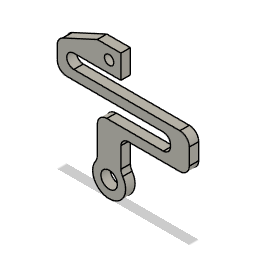
_VEER.274ef9a5-93d1-4273-a178-3e04e85e3114 (Autodesk Fusion 360 design; units mm, degrees)
Autodesk Fusion 360 part; units mm, degrees
sketch "Sketch1" plane through (0, 0, 0) normal (0, 0, 1) x (1, 0, 0)
  line L0 (2.5, 19.5) -> (2.5, 24.5)
  line L1 (-8.5, 21.7171) -> (-8.5, 21.7081)
  line L2 (2.5, 19.5) -> (2.5, 24.5)
  circle A0 centre (0, 0) radius 1.75
  circle A1 centre (0, 22) radius 1
  line L3 (0, 19.5812) -> (0, -19.5812) construction
  line L4 (2.5, 0) -> (-2.5, 0)
  line L5 (-2.5, 3.1623) -> (-2.5, 9)
  line L6 (-0.5, 11) -> (2.5, 11)
  line L7 (2.5, 7.5) -> (2.5, 3.1623)
  line L8 (2.5, 0) -> (-2.5, 11) construction
  line L9 (-2.5, 0) -> (2.5, 11) construction
  line L10 (-0.5, 11) -> (11.5, 11)
  line L11 (17, 11) -> (17, 9)
  line L12 (15, 9) -> (4, 9)
  line L13 (-2.5, 9) -> (-2.5, 11)
  line L14 (17, 9) -> (13, 9)
  line L15 (13, 12.5) -> (13, 13)
  line L16 (13, 16.5) -> (17, 16.5)
  line L17 (17, 14.5) -> (17, 11)
  line L18 (15, 16.5) -> (-7.5, 16.5)
  line L19 (-9, 14.5) -> (11.5, 14.5)
  line L20 (17, 14.5) -> (17, 16.5)
  line L21 (2.5, 19.5) -> (-2.5, 19.5)
  line L22 (-2.5, 19.5) -> (-2.5, 24.5)
  line L23 (-2.5, 24.5) -> (2.5, 24.5)
  line L24 (2.5, 24.5) -> (2.5, 19.5)
  line L25 (2.5, 19.5) -> (-2.5, 24.5) construction
  line L26 (-2.5, 19.5) -> (2.5, 24.5) construction
  line L27 (2.5, 19.5) -> (-7.5, 19.5)
  line L28 (-2.5, 21.5) -> (2.5, 21.5)
  line L29 (2.5, 21.5) -> (2.5, 19.5)
  line L30 (-9, 18) -> (-11, 18)
  line L31 (-11, 16.5) -> (-11, 19.2973)
  line L32 (-2.5, 24.5) -> (-9.8381, 21.1132)
  arc A2 (-7.5, 19.5) -> (-9, 18) centre (-7.5, 18) ccw
  arc A3 (-9, 18) -> (-7.5, 16.5) centre (-7.5, 18) ccw
  arc A4 (13, 13) -> (11.5, 14.5) centre (11.5, 13) ccw
  arc A5 (11.5, 11) -> (13, 12.5) centre (11.5, 12.5) ccw
  arc A6 (4, 9) -> (2.5, 7.5) centre (4, 7.5) ccw
  arc A7 (-11, 16.5) -> (-9, 14.5) centre (-9, 16.5) ccw
  arc A8 (17, 14.5) -> (15, 16.5) centre (15, 14.5) ccw
  arc A9 (15, 9) -> (17, 11) centre (15, 11) ccw
  arc A10 (-9.8381, 21.1132) -> (-11, 19.2973) centre (-9, 19.2973) ccw
  arc A11 (-0.5, 11) -> (-2.5, 9) centre (-0.5, 9) ccw
  arc A12 (-0.9716, 3.3624) -> (-2.5, 2.4495) centre (0, 0) ccw
  arc A13 (-2.8636, 2.0124) -> (2.8636, 2.0124) centre (0, 0) ccw
  arc A14 (0.9716, 3.3624) -> (-0.9716, 3.3624) centre (0, 0) ccw
  arc A15 (2.5, 2.4495) -> (0.9716, 3.3624) centre (0, 0) ccw
  arc A16 (2.5, 3.1623) -> (2.8636, 2.0124) centre (4.5, 3.1623) ccw
  arc A17 (-2.8636, 2.0124) -> (-2.5, 3.1623) centre (-4.5, 3.1623) ccw
  point P0 (0, 5.5)
  point P1 (0, 5.5)
  point P2 (0, 22)
  dimension "d1" = 3.5
  dimension "d5" = 2
  dimension "d8" = 22
  dimension "d12" = 5
  dimension "d16" = 7
  dimension "d19" = 5
  dimension "d20" = 11
  dimension "d21" = 19.5
  dimension "d22" = 2
  dimension "d23" = 4
  dimension "d24" = 7.5
  dimension "d26" = 2
  dimension "d27" = 5
  dimension "d28" = 5
  dimension "d30" = 2
  dimension "d32" = 1.5
  dimension "d33" = 2
  dimension "d34" = 2
  constraint coincident P2 L3
  constraint vertical L3
  constraint concentric A0 A13
  constraint coincident A0.centre A12.centre
  constraint coincident L3 P1
  constraint horizontal L4
  constraint perpendicular L4 L5
  constraint parallel L4 L6
  constraint parallel L5 L7
  constraint coincident L8 P1
  constraint coincident L9 P1
  constraint midpoint A0.centre L4
  constraint horizontal L10
  constraint vertical L11
  constraint horizontal L12
  constraint vertical L13
  constraint horizontal L14
  constraint vertical L15
  constraint horizontal L16
  constraint vertical L17
  constraint horizontal L18
  constraint horizontal L19
  constraint vertical L20
  constraint horizontal L21
  constraint perpendicular L21 L22
  constraint parallel L21 L23
  constraint parallel L22 L24
  constraint coincident L25 P2
  constraint coincident L26 P2
  constraint coincident P2 A1.centre
  constraint horizontal L27
  constraint horizontal L28
  constraint vertical L29
  constraint horizontal L30
  constraint vertical L31
  constraint tangent L27 A2
  constraint tangent L18 A3
  constraint equal A2 A3
  constraint coincident L30.start A2.end
  constraint coincident L17.start L19
  constraint coincident L16.start L15
  constraint tangent L19 A4
  constraint tangent L15 A4
  constraint equal A2 A4
  constraint coincident L14.end L15
  constraint coincident L11.start L10
  constraint tangent L15 A5
  constraint tangent L10 A5
  constraint equal A2 A5
  constraint coincident L6.end L7
  constraint coincident L5.end L12
  constraint tangent L7 A6
  constraint tangent L12 A6
  constraint equal A2 A6
  constraint tangent L19 A7
  constraint coincident L16.end L18
  constraint coincident L16.end L17
  constraint tangent L18 A8
  constraint tangent L17 A8
  constraint equal A7 A8
  constraint coincident L11.end L17
  constraint coincident L11.end L12
  constraint tangent L17 A9
  constraint tangent L12 A9
  constraint equal A7 A9
  constraint tangent L32 A10
  constraint tangent L31 A10
  constraint equal A7 A10
  constraint coincident L8.end L6
  constraint coincident L8.end L5
  constraint tangent L6 A11
  constraint tangent L5 A11
  constraint equal A7 A11
  constraint coincident L30.end L31
  constraint coincident L22 L28.start
  constraint coincident L9 A12.start
  constraint coincident L5 A12.end
  constraint concentric A12 A13
  constraint coincident L7 A15.start
  constraint coincident L8 A14.start
  constraint concentric A13 A14
  constraint concentric A13 A15
  constraint tangent A13 A16
  constraint tangent L7 A16
  constraint tangent A13 A17
  constraint tangent L5 A17
  constraint equal A16 A17
  measures "d1" diameter of A0
  measures "d5" diameter of A1
  measures "d8" distance of A0.centre P2
  measures "d12" distance of L0.start L0.end
  measures "d16" diameter of A13
  measures "d19" distance of L8.end L6.end
  measures "d20" distance of L4.end L8.end
  measures "d21" distance of L8.end L11.start
  measures "d22" distance of L8.end L5.end
  measures "d23" distance of L11.end L14.end
  measures "d24" distance of L11.end L16.end
  measures "d26" distance of L16.end L17.start
  measures "d27" distance of L22.end L0.end
  measures "d28" distance of L21.end L22.end
  measures "d30" distance of L0.start L28.end
  measures "d32" radius of A2
  measures "d33" radius of A7
  measures "d34" radius of A16
extrude "Extrude1" add sketch "Sketch1" along normal blind 2 contours L0 L2 A1 L21 L22 L24 L27 L28 L29 | L0 L2 A1 L22 L23 L24 L28 | L22 L27 L30 L31 L32 A2 A10 | L5 L6 L7 L10 L12 L14 L15 L16 L17 L18 L19 L30 L31 A3 A4 A5 A6 A7 A8 A9 A11 A13 A16 A17
